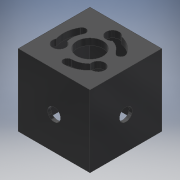
# Autodesk Inventor part: Case1
Saved by Autodesk Inventor 2019 (Build 230136000, 136)
## iProperties
Created: 2019-06-21
Part Number: Case1
Material: Steel, Mild, Welded
Document SubType Name: Modeling
Designer: hecto
Density: 7.85 g/cm^3
Appearance: Smooth - Dark Gray
Author: hecto
Autodesk Inventor part; units mm, degrees
ref_plane "YZ Plane" through (0, 0, 0) normal (1, 0, 0) x (0, 1, 0)
ref_plane "XZ Plane" through (0, 0, 0) normal (0, 1, 0) x (-1, 0, 0)
ref_plane "XY Plane" through (0, 0, 0) normal (0, 0, 1) x (1, 0, 0)
sketch "Sketch1" plane through (0, 0, 0) normal (0, 1, 0) x (-1, 0, 0)
  line L0 (0, -34.641) -> (30, 17.3205) construction
  line L1 (30, 17.3205) -> (-30, 17.3205) construction
  line L2 (-30, 17.3205) -> (0, -34.641) construction
  circle A0 centre (0, 0) radius 34.641 construction
  circle A1 centre (0, -34.641) radius 10
  circle A2 centre (-30, 17.3205) radius 10
  circle A3 centre (30, 17.3205) radius 10
  circle A4 centre (0, 0) radius 20
  line L3 (55, -55) -> (-55, -55)
  line L4 (-55, -55) -> (-55, 55)
  line L5 (-55, 55) -> (55, 55)
  line L6 (55, 55) -> (55, -55)
  circle A5 centre (0, 0) radius 45 construction
  point P0 (0, -55)
  point P1 (55, 0)
  dimension "d0" = 60
  dimension "d1" = 20
  dimension "d2" = 40
  dimension "d3" = 90
  dimension "d4" = 55
  constraints: 14 end point, 6 centre point, 6 coincident, 3 equal length, 2 equal radius, 2 horizontal, 2 midpoint, 2 parallel, 2 point on circle, 2 vertical alignment, 1 horizontal alignment, 1 perpendicular
  measures "d0" distance of L1.end L0.start
  measures "d1" diameter of A1
  measures "d2" diameter of A4
  measures "d3" diameter of A5
  measures "d4" distance from line of L6 point (0, 0)
extrude "Extrusion1" add sketch "Sketch1" against normal blind 110
sketch "Sketch2" plane through (0, 0, 0) normal (0, 1, 0) x (1, 0, 0)
  circle A0 centre (0, 0) radius 20 projected
  circle A1 centre (-30, -17.3205) radius 10 projected
  circle A2 centre (30, -17.3205) radius 10 projected
  circle A3 centre (0, 34.641) radius 10 projected
  line L0 (-55, 55) -> (55, 55) projected
  line L1 (-55, -55) -> (-55, 55) projected
  line L2 (55, -55) -> (-55, -55) projected
  line L3 (55, 55) -> (55, -55) projected
  circle A4 centre (0, 34.641) radius 6.25
  circle A5 centre (-30, 17.3205) radius 6.25
  circle A6 centre (-30, -17.3205) radius 6.25
  circle A7 centre (0, -34.641) radius 6.25
  circle A8 centre (30, -17.3205) radius 6.25
  circle A9 centre (30, 17.3205) radius 6.25
  arc A10 (-35.4127, 20.4455) -> (-35.4127, -20.4455) centre (0, 0) ccw
  arc A11 (-24.5873, 14.1955) -> (-24.5873, -14.1955) centre (0, 0) ccw
  arc A12 (0, -40.891) -> (35.4127, -20.4455) centre (0, 0) ccw
  arc A13 (35.4127, 20.4455) -> (0, 40.891) centre (0, 0) ccw
  arc A14 (0, -28.391) -> (24.5873, -14.1955) centre (0, 0) ccw
  arc A15 (24.5873, 14.1955) -> (0, 28.391) centre (0, 0) ccw
  dimension "d7" = 12.5
  dimension "d10" = 360
  constraints: 24 point on circle, 12 centre point, 6 tangent, 3 coincident, 13 other
  measures "d7" diameter of A4
extrude "Extrusion2" cut sketch "Sketch2" against normal through all contours A11 A6 A10 A1 | A1 A10 A5 A11 | A5 | A14 A8 A12 A2 | A2 A12 A7 A14 | A7 | A3 A15 A4 A13 | A3 A13 A9 A15 | A9 picked at (-34.5635, -9.9186) picked at (25.4365, -24.7224) picked at (8.6846, 33.9839)
sketch "Sketch3" plane through (0, -110, 0) normal (0, -1, 0) x (1, 0, 0)
  line L0 (-55, -55) -> (55, -55) projected
  line L1 (55, -55) -> (55, 55) projected
  line L2 (55, 55) -> (-55, 55) projected
  line L3 (-55, 55) -> (-55, -55) projected
  arc A0 (7.0121, -27.5115) -> (24.5873, -14.1955) centre (0, 0) ccw projected
  arc A1 (35.4127, -20.4455) -> (24.5873, -14.1955) centre (30, -17.3205) ccw projected
  arc A2 (8.4355, -40.0115) -> (35.4127, -20.4455) centre (0, 0) ccw projected
  arc A3 (7.0121, -27.5115) -> (8.4355, -40.0115) centre (0, -34.641) ccw projected
  arc A4 (20.3196, 19.8284) -> (0, 28.391) centre (0, 0) ccw projected
  arc A5 (0, 40.891) -> (0, 28.391) centre (0, 34.641) ccw projected
  arc A6 (30.4332, 27.3111) -> (0, 40.891) centre (0, 0) ccw projected
  arc A7 (20.3196, 19.8284) -> (30.4332, 27.3111) centre (30, 17.3205) ccw projected
  arc A8 (-27.3317, 7.6831) -> (-24.5873, -14.1955) centre (0, 0) ccw projected
  arc A9 (-35.4127, -20.4455) -> (-24.5873, -14.1955) centre (-30, -17.3205) ccw projected
  arc A10 (-38.8687, 12.7003) -> (-35.4127, -20.4455) centre (0, 0) ccw projected
  arc A11 (-27.3317, 7.6831) -> (-38.8687, 12.7003) centre (-30, 17.3205) ccw projected
  circle A12 centre (0, 0) radius 20 projected
  line L4 (-50, 50) -> (50, 50)
  line L5 (50, 50) -> (50, -50)
  line L6 (50, -50) -> (-50, -50)
  line L7 (-50, -50) -> (-50, 50)
  dimension "d14" = 5
  constraints: 8 end point, 3 other
  measures "d14" distance between parallel lines of L2 L4
extrude "Extrusion3" cut sketch "Sketch3" against normal blind 100 contours A0 A1 A2 A3 | A4 A5 A6 A7 | A8 A9 A10 A11 | A12 | L4 L5 L6 L7
sketch "Sketch5" plane through (55, 0, -55) normal (0, 0, -1) x (-1, 0, 0)
  circle A0 centre (55, -60) radius 10
  line L0 (110, -110) -> (0, -110) projected
  line L1 (110, 0) -> (0, 0) projected
  point P0 (55, 0)
  point P1 (55, -110)
  dimension "d17" = 60
  dimension "d20" = 20
  constraints: 1 centre point, 1 midpoint, 1 vertical alignment
  measures "d17" distance from line of L1 A0.centre
  measures "d20" diameter of A0
extrude "Extrusion4" cut sketch "Sketch5" against normal through all
sketch "Sketch6" plane through (55, 0, 55) normal (1, 0, 0) x (0, 0, -1)
  circle A0 centre (55, -60) radius 10
  line L0 (110, -110) -> (0, -110) projected
  line L1 (110, 0) -> (0, 0) projected
  point P0 (55, 0)
  point P1 (55, -110)
  dimension "d21" = 20
  dimension "d22" = 60
  constraints: 1 centre point, 1 midpoint, 1 vertical alignment
  measures "d21" diameter of A0
  measures "d22" distance from line of L1 A0.centre
extrude "Extrusion5" cut sketch "Sketch6" against normal up to next
sketch "Sketch7" plane through (-50, -110, 50) normal (1, 0, 0) x (0, 0, -1)
  circle A0 centre (90, 15) radius 5
  line L0 (105, 110) -> (105, 0) projected
  line L1 (-5, 0) -> (105, 0) projected
  point P0 (50, 110)
  dimension "d25" = 10
  dimension "d26" = 15
  dimension "d27" = 15
  constraints: 1 centre point
  measures "d25" diameter of A0
  measures "d26" distance from line of L0 A0.centre
  measures "d27" distance from line of L1 A0.centre
extrude "Extrusion6" cut sketch "Sketch7" against normal through all
body "Solid1"
